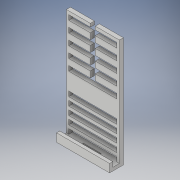
# Autodesk Inventor part: Kirtiman phone charger design
Saved by Autodesk Inventor 2019 (Build 230136000, 136)
## iProperties
Created: 2020-04-05
Part Number: Kirtiman phone charger design
Material: Generic
Document SubType Name: Modeling
Designer: Manoj
Density: 1 g/cm^3
Appearance: Default
Author: Manoj
Autodesk Inventor part; units mm, degrees
ref_plane "YZ Plane" through (0, 0, 0) normal (1, 0, 0) x (0, 1, 0)
ref_plane "XZ Plane" through (0, 0, 0) normal (0, 1, 0) x (-1, 0, 0)
ref_plane "XY Plane" through (0, 0, 0) normal (0, 0, 1) x (1, 0, 0)
sketch "Sketch1" plane through (0, 0, 0) normal (0, 0, 1) x (1, 0, 0)
  line L0 (-32.5, 75) -> (32.5, 75)
  line L1 (32.5, 75) -> (32.5, -60)
  line L2 (32.5, -60) -> (-32.5, -60)
  line L3 (-32.5, -60) -> (-32.5, 75)
  point P0 (0, 0)
  dimension "d0" = 65
  dimension "d1" = 135
  dimension "d2" = 32.5
  dimension "d3" = 60
  constraints: 8 end point, 2 parallel, 1 horizontal, 1 perpendicular
  measures "d0" distance of L1.end L2.end
  measures "d1" distance of L0.end L1.end
  measures "d2" distance from line of L1 point (0, 0)
  measures "d3" distance from line of L2 point (0, 0)
extrude "Extrusion1" add sketch "Sketch1" along normal blind 5
sketch "Sketch2" plane through (0, 0, 5) normal (0, 0, 1) x (1, 0, 0)
  line L0 (-32.5, 75) -> (-32.5, -60) projected
  line L1 (-32.5, -60) -> (32.5, -60) projected
  line L2 (-32.5, -56) -> (32.5, -56)
  line L3 (32.5, -56) -> (32.5, -60)
  line L4 (32.5, -60) -> (-32.5, -60)
  line L5 (-32.5, -60) -> (-32.5, -56)
  point P0 (0, 0)
  dimension "d6" = 4
  constraints: 8 end point, 2 parallel, 1 horizontal, 1 perpendicular, 1 point on line
  measures "d6" distance between parallel lines of L1 L2
extrude "Extrusion2" add sketch "Sketch2" along normal blind 8
sketch "Sketch3" plane through (0, 0, 13) normal (0, 0, 1) x (1, 0, 0)
  line L0 (-32.5, -60) -> (-32.5, 75) projected
  line L1 (32.5, 75) -> (32.5, -60) projected
  line L2 (-32.5, -50) -> (32.5, -50)
  line L3 (32.5, -50) -> (32.5, -60)
  line L4 (32.5, -60) -> (-32.5, -60)
  line L5 (-32.5, -60) -> (-32.5, -50)
  point P0 (0, 0)
  dimension "d9" = 10
  constraints: 8 end point, 2 parallel, 1 horizontal, 1 perpendicular, 1 point on line
  measures "d9" distance between parallel lines of L4 L2
extrude "Extrusion3" add sketch "Sketch3" along normal blind 4
sketch "Sketch4" plane through (0, 0, 5) normal (0, 0, 1) x (1, 0, 0)
  line L0 (-32.5, -60) -> (-32.5, 75) projected
  line L1 (32.5, 75) -> (32.5, -60) projected
  line L2 (32.5, 75) -> (32.5, 71)
  line L3 (-32.5, 71) -> (-32.5, 75)
  point P0 (0, 0)
  constraints: 4 end point, 1 parallel, 1 point on line
sketch "Sketch6" plane through (-32.5, -60, 0) normal (0, -1, 0) x (1, 0, 0)
  line L0 (65, 13) -> (0, 13) projected
  line L1 (21.6667, 13) -> (43.3333, 13)
  line L2 (43.3333, 13) -> (43.3333, 5.6667)
  line L3 (43.3333, 5.6667) -> (21.6667, 5.6667)
  line L4 (21.6667, 5.6667) -> (21.6667, 13)
  line L5 (65, 0) -> (65, 17) projected
  line L6 (0, 0) -> (0, 17) projected
  line L7 (65, 0) -> (0, 0) projected
  line L8 (0, 17) -> (65, 17) projected
  point P0 (32.5, 0)
  dimension "d18" = 21.6667
  dimension "d19" = 21.6667
  dimension "d20" = 5.6667
  dimension "d21" = 4
  constraints: 8 end point, 2 parallel, 1 horizontal, 1 perpendicular, 1 point on line
  measures "d18" distance between parallel lines of L5 L2
  measures "d19" distance between parallel lines of L6 L4
  measures "d20" distance between parallel lines of L3 L7
  measures "d21" distance between parallel lines of L8 L0
extrude "Extrusion6" cut sketch "Sketch6" against normal blind 206 contours L2 L3 L4 L0
sketch "Sketch7" plane through (0, 0, 0) normal (0, 0, -1) x (-1, 0, 0)
  line L0 (32.5, -56) -> (-32.5, -56) projected
  line L1 (29.5, -56) -> (-29.5, -56)
  line L2 (-29.5, -56) -> (-29.5, -50)
  line L3 (-32.5, -50) -> (32.5, -50) projected
  line L4 (-29.5, -50) -> (29.5, -50)
  line L5 (29.5, -50) -> (29.5, -56)
  line L6 (32.5, -60) -> (32.5, 75) projected
  line L7 (-32.5, 75) -> (-32.5, -60) projected
  line L8 (29.5, -46) -> (-29.5, -46)
  line L9 (-29.5, -46) -> (-29.5, -40)
  line L10 (-29.5, -40) -> (29.5, -40)
  line L11 (29.5, -40) -> (29.5, -46)
  line L12 (29.5, -36) -> (-29.5, -36)
  line L13 (-29.5, -36) -> (-29.5, -30)
  line L14 (-29.5, -30) -> (29.5, -30)
  line L15 (29.5, -30) -> (29.5, -36)
  line L16 (29.5, -26) -> (-29.5, -26)
  line L17 (-29.5, -26) -> (-29.5, -20)
  line L18 (-29.5, -20) -> (29.5, -20)
  line L19 (29.5, -20) -> (29.5, -26)
  line L20 (29.5, -16) -> (-29.5, -16)
  line L21 (-29.5, -16) -> (-29.5, -10)
  line L22 (-29.5, -10) -> (29.5, -10)
  line L23 (29.5, -10) -> (29.5, -16)
  line L24 (32.5, 65) -> (-32.5, 65) projected
  line L25 (-32.5, 71) -> (32.5, 71) projected
  line L26 (29.5, 65) -> (-29.5, 65)
  line L27 (-29.5, 65) -> (-29.5, 71)
  line L28 (-29.5, 71) -> (29.5, 71)
  line L29 (29.5, 71) -> (29.5, 65)
  line L30 (29.5, 51.5) -> (-29.5, 51.5)
  line L31 (29.5, 57.5) -> (29.5, 51.5)
  line L32 (-29.5, 57.5) -> (29.5, 57.5)
  line L33 (-29.5, 51.5) -> (-29.5, 57.5)
  line L34 (29.5, 38) -> (-29.5, 38)
  line L35 (29.5, 44) -> (29.5, 38)
  line L36 (-29.5, 44) -> (29.5, 44)
  line L37 (-29.5, 38) -> (-29.5, 44)
  line L38 (29.5, 24.5) -> (-29.5, 24.5)
  line L39 (29.5, 30.5) -> (29.5, 24.5)
  line L40 (-29.5, 30.5) -> (29.5, 30.5)
  line L41 (-29.5, 24.5) -> (-29.5, 30.5)
  line L42 (29.5, 11) -> (-29.5, 11)
  line L43 (29.5, 17) -> (29.5, 11)
  line L44 (-29.5, 17) -> (29.5, 17)
  line L45 (-29.5, 11) -> (-29.5, 17)
  point P0 (0, 0)
  dimension "d24" = 3
  dimension "d25" = 3
  dimension "d30" = 10
  dimension "d35" = 3
  dimension "d36" = 3
  dimension "d39" = 13.5
  constraints: 80 end point, 6 point on line, 3 perpendicular, 2 parallel, 2 vertical, 1 horizontal, 64 other
  measures "d24" distance between parallel lines of L6 L5
  measures "d25" distance between parallel lines of L7 L2
  measures "d30" distance of L1.start L8.start
  measures "d35" distance between parallel lines of L7 L27
  measures "d36" distance between parallel lines of L29 L6
  measures "d39" distance of L26.start L30.start
extrude "Extrusion7" cut sketch "Sketch7" against normal up to surface (5 mm away) contours L0 L2 L3 L5
extrude "Extrusion8" cut sketch "Sketch7" against normal up to surface (5 mm away) contours L24 L27 L25 L29 | L8 L9 L10 L11 | L12 L13 L14 L15 | L16 L17 L18 L19 | L20 L21 L22 L23 | L30 L33 L32 L31 | L34 L37 L36 L35 | L38 L41 L40 L39 | L42 L45 L44 L43
sketch "Sketch8" plane through (0, 0, 0) normal (0, 0, -1) x (-1, 0, 0)
  line L0 (32.5, 75) -> (-32.5, 75) projected
  line L1 (-29.5, 11) -> (29.5, 11) projected
  line L2 (-3, 75) -> (3, 75)
  line L3 (3, 75) -> (3, 11)
  line L4 (3, 11) -> (-3, 11)
  line L5 (-3, 11) -> (-3, 75)
  line L6 (32.5, -60) -> (32.5, 75) projected
  line L7 (-32.5, 75) -> (-32.5, -60) projected
  point P0 (0, 0)
  dimension "d46" = 29.5
  dimension "d47" = 29.5
  constraints: 8 end point, 2 parallel, 2 point on line, 1 horizontal, 1 perpendicular
  measures "d46" distance between parallel lines of L6 L3
  measures "d47" distance between parallel lines of L7 L5
extrude "Extrusion9" cut sketch "Sketch8" against normal blind 206
body "Solid1"
